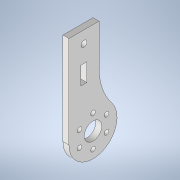
# Autodesk Inventor part: Brazo3
Saved by Autodesk Inventor 2022 (Build 260153000, 153)
## iProperties
Created: 2021-09-13
Part Number: Brazo3
Material: Generic
Document SubType Name: Modeling
Designer: Administrador
Density: 1 g/cm^3
Appearance: Default
Author: Administrador
Autodesk Inventor part; units mm, degrees
ref_plane "YZ Plane" through (0, 0, 0) normal (1, 0, 0) x (0, 1, 0)
ref_plane "XZ Plane" through (0, 0, 0) normal (0, 1, 0) x (-1, 0, 0)
ref_plane "XY Plane" through (0, 0, 0) normal (0, 0, 1) x (1, 0, 0)
sketch "Sketch1" plane through (0, 0, 0) normal (1, 0, 0) x (0, 1, 0)
  arc A0 (0.0036, 12) -> (0.0036, -12) centre (0.0036, 0) ccw
  circle A1 centre (0.0036, 0) radius 4.375
  circle A2 centre (0.0036, 0) radius 9 construction
  line L0 (-11.9964, 0) -> (0.0036, 0) construction
  line L1 (-8.9964, 0) -> (-7.7964, 0)
  circle A3 centre (-7.7964, 0) radius 1.2
  circle A4 centre (-3.8964, -6.755) radius 1.2
  circle A5 centre (3.9036, -6.755) radius 1.2
  circle A6 centre (7.8036, 0) radius 1.2
  circle A7 centre (3.9036, 6.755) radius 1.2
  circle A8 centre (-3.8964, 6.755) radius 1.2
  line L2 (-11.9964, 0) -> (33.0036, 0) construction
  line L3 (-11.9964, 37.6945) -> (46.0036, 37.6945) construction
  line L4 (0.0036, 12) -> (46.0036, 12)
  line L5 (46.0036, 12) -> (46.0036, -3)
  arc A9 (0.0036, -12) -> (7.4266, -9.4286) centre (0.0036, 0) ccw
  arc A10 (25.9843, -3) -> (7.4266, -9.4286) centre (25.9843, -33) ccw
  line L6 (25.9843, -3) -> (46.0036, -3)
  circle A11 centre (40.0036, 4.5) radius 1.5
  line L7 (31.5036, 6) -> (22.5036, 6)
  line L8 (22.5036, 6) -> (22.5036, 3)
  line L9 (22.5036, 3) -> (31.5036, 3)
  line L10 (31.5036, 3) -> (31.5036, 6)
  point P0 (1.5, 26.1095)
  point P1 (22.5, 26.1095)
  point P2 (-4.4964, -7.7942)
  point P3 (4.5036, -7.7942)
  point P4 (9.0036, 0)
  point P5 (4.5036, 7.7942)
  point P6 (-4.4964, 7.7942)
  point P7 (11.6225, -3)
  dimension "d4" = 18
  dimension "d2" = 24
  dimension "d3" = 8.75
  dimension "d5" = 1.2
  dimension "d7" = 360
  dimension "d8" = 45
  dimension "d12" = 12
  dimension "d15" = 58
  dimension "d16" = 15
  dimension "d18" = 30
  dimension "d22" = 3
  dimension "d23" = 6
  dimension "d28" = 7.5
  dimension "d29" = 15
  dimension "d31" = 9
  dimension "d32" = 3
  constraints: 22 end point, 8 point on circle, 5 centre point, 4 horizontal, 3 coincident, 3 horizontal alignment, 2 parallel, 2 point on line, 2 tangent, 1 perpendicular, 1 vertical, 37 other
  measures "d2" diameter of A0
  measures "d3" diameter of A1
  measures "d5" distance of L1.start L1.end
  measures "d8" distance of L0.start L2.end
  measures "d12" distance of L0.start A0.centre
  measures "d15" distance of L3.start L3.end
  measures "d16" distance of L4.end L5.end
  measures "d18" radius of A10
  measures "d22" diameter of A11
  measures "d23" distance from line of L5 A11.centre
  measures "d28" distance from line of L6 A11.centre
  measures "d29" distance between parallel lines of L6 L4
  measures "d31" distance of L9.end L8.end
  measures "d32" distance of L8.end L7.end
extrude "Extrusion1" add sketch "Sketch1" along normal blind 3
body "Solid1"
